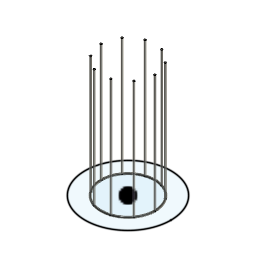
Installation Sketch v1 (Autodesk Fusion 360 design; units mm, degrees)
Autodesk Fusion 360 part; units mm, degrees
sketch "Skizze1" plane through (0, 0, 0) normal (0, 0, 1) x (1, 0, 0)
  circle A0 centre (0, 0) radius 250
  dimension "d1" = 500
  constraint coincident A0.centre origin
  measures "d1" diameter of A0
sketch "Skizze2" plane through (0, 0, 0) normal (0, 0, 1) x (1, 0, 0)
  circle A0 centre (0, 0) radius 400
  dimension "d2" = 800
  constraint coincident A0.centre origin
  measures "d2" diameter of A0
pipe "Leitung1" add diameter 20 path "Skizze1" along A0 makes body 1
sketch "Skizze3" plane through (0, 0, 0) normal (0, 0, 1) x (1, 0, 0)
  circle A0 centre (-250, 0) radius 9
  circle A1 centre (0, 0) radius 250
  dimension "d7" = 18
  constraint coincident A0.centre A1
  constraint horizontal A0.centre A1.centre
  measures "d7" diameter of A0
extrude "Extrusion1" add sketch "Skizze3" along normal blind 1100 separate body contours A0 A1 | A0 A1 picked at (-246.988, 0) picked at (-252.988, 0) makes body 2
pattern_circular "C-Anordnung1" count 10 over 360 about axis through (0, 0, 1.75) along (0, 0, 1) of bodies 2 makes body 3 at (-211.2357, -146.3686, 733.3333) makes body 4 at (-86.2541, -237.7079, 733.3333) makes body 5 at (85.7983, -240.5923, 733.3333) makes body 6 at (208.5406, -140.5056, 733.3333) makes body 7 at (257.7671, 4.5467, 733.3333) makes body 8 at (211.2357, 146.3686, 733.3333) makes body 9 at (86.2541, 237.7079, 733.3333) makes body 10 at (-85.7983, 240.5923, 733.3333) makes body 11 at (-208.5406, 140.5056, 733.3333)
